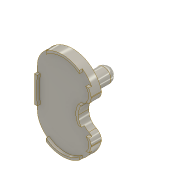
# Autodesk Inventor part: 1
Saved by Autodesk Inventor 2017 (Build 210142000, 142)
## iProperties
Created: 2020-04-05
Part Number: 1
Material: Tytan 6Al-4V
Document SubType Name: Modeling
Designer: Kinga Nowak
Density: 4.43 g/cm^3
Appearance: Tytan — polerowany
Authority: dr Marta Kiel-Jamrozik
Checked By: dr Marta Kiel-Jamrozik
Mfg Approved By: dr Marta Kiel-Jarmozik
Description: Endoproteza stawu kolanowego
Project: część piszczelowa
Author: Kinga Nowak
Autodesk Inventor part; units mm, degrees
ref_plane "YZ Plane" through (0, 0, 0) normal (1, 0, 0) x (0, 1, 0)
ref_plane "XZ Plane" through (0, 0, 0) normal (0, 1, 0) x (-1, 0, 0)
sketch "Szkic1" plane through (0, 0, 0) normal (0, 1, 0) x (-1, 0, 0)
  line L0 (-4, -50.1202) -> (-4, -37.2024)
  line L1 (-42.5, -51.8732) -> (-42.5, -51.3513)
  line L2 (-4, -38) -> (-4, -50.1202)
  arc A0 (-38.9822, -45.8888) -> (-34, -38.0004) centre (-42.4987, -38.1503) ccw
  line L3 (-42.5, -51.3513) -> (-42.5, -51.8732)
  arc A1 (-34, -38.0004) -> (-34.0517, -37.2023) centre (-42.4987, -38.1503) ccw
  arc A2 (-38.9822, -45.8888) -> (-42.5, -51.3513) centre (-36.5, -51.3513) ccw
  arc A3 (-42.5, -51.8732) -> (-6.8354, -58.8964) centre (-23.0549, -47.1948) ccw
  arc A4 (-6.8354, -58.8964) -> (-4, -50.1202) centre (-19, -50.1202) ccw
  line L4 (-42.5, -51.3513) -> (-42.5, -51.8732)
  line L5 (-4, -24.2847) -> (-4, -37.2024)
  line L6 (-42.5, -22.5011) -> (-42.5, -23.0533)
  line L7 (-4, -36.4049) -> (-4, -24.2847)
  arc A5 (-34, -36.4047) -> (-38.9822, -28.5157) centre (-42.4987, -36.2542) ccw
  line L8 (-42.5, -23.0533) -> (-42.5, -22.5011)
  arc A6 (-34.0517, -37.2023) -> (-34, -36.4047) centre (-42.4987, -36.2542) ccw
  arc A7 (-42.5, -23.0533) -> (-38.9822, -28.5157) centre (-36.5, -23.0533) ccw
  arc A8 (-6.8187, -15.5316) -> (-42.5, -22.5011) centre (-23.0604, -27.2024) ccw
  arc A9 (-4, -24.2847) -> (-6.8187, -15.5316) centre (-19, -24.2847) ccw
  line L9 (-42.5, -23.0533) -> (-42.5, -22.5011)
  line L10 (-12, -10.5391) -> (-12, -12.5391)
  line L11 (-34.5, -10.7971) -> (-34.5, -12.7971)
  arc A10 (-12, -12.5391) -> (-34.5, -12.7971) centre (-23.0889, -26.7178) ccw
  line L12 (-11.9997, -63.8616) -> (-11.9997, -61.8657)
  line L13 (-34.5004, -63.596) -> (-34.5004, -61.6077)
  arc A11 (-34.5004, -61.6077) -> (-11.9997, -61.8657) centre (-23.0889, -47.6872) ccw
  line L14 (-35.8952, -43.5023) -> (-33.8952, -43.5023)
  line L15 (-35.8952, -30.9023) -> (-33.8952, -30.9023)
  arc A12 (-33.8952, -43.5023) -> (-33.8952, -30.9023) centre (-44.1084, -37.2023) ccw
  line L16 (-4, -28) -> (-6, -28)
  line L17 (-6, -46) -> (-4, -46)
  arc A13 (-6, -46) -> (-6, -28) centre (-89.405, -37) ccw
  line L18 (-40.8175, -18) -> (-38.8175, -18)
  line L19 (-40.8176, -27.2196) -> (-38.8176, -27.2198)
  arc A14 (-38.8175, -18) -> (-38.9822, -27.2198) centre (-34.316, -22.6918) ccw
  line L20 (-41.0122, -56.0002) -> (-39.0216, -56.0002)
  line L21 (-39.0216, -56.0002) -> (-41.0122, -56.0002)
  line L22 (-41.0216, -47.4073) -> (-39.0216, -47.4076)
  arc A15 (-39.0216, -47.4076) -> (-39.0216, -56.0002) centre (-35.5308, -51.7039) ccw
  line L23 (-19, -7.6189) -> (11, -7.6189) construction
  point P0 (0, 0)
  point P1 (-42.5001, -29.6503)
  point P2 (-4, -22.2491)
  point P3 (-23.0549, -67.1948)
  point P4 (-23.0549, -67.1948)
  point P5 (-42.5, -44.7542)
  point P6 (-23.0604, -7.2024)
  point P7 (-23.0604, -7.2024)
  dimension "d12" = 15
  dimension "d13" = 30
  dimension "d14" = 6
  dimension "d15" = 20
  dimension "d21" = 38.5
  dimension "d53" = 2
  constraints: 49 point on circle, 48 end point, 16 centre point, 4 horizontal, 4 point on line, 4 tangent, 4 vertical, 2 coincident, 2 parallel, 1 collinear, 1 perpendicular, 5 other
  measures "d12" radius of A4
  measures "d13" distance from line of L0 A0.end
  measures "d14" radius of A2
  measures "d15" radius of A3
  measures "d21" distance from line of L1.end L2
  measures "d53" distance of L18.start L18.end
extrude "Wyciągnięcie proste1" add sketch "Szkic1" along normal blind 5
extrude "Wyciągnięcie proste2" add sketch "Szkic1" against normal blind 2 contours L17 A13 L16 L5 L0 | A3 L13 A11 L12 | A3 L1 A2 L22 A15 L20 | L10 A10 L11 A8 | L18 A14 L19 A7 L6 A8 | A0 A1 A6 A5 L15 A12 L14
sketch "Szkic5" plane through (0, 5, 0) normal (0, 1, 0) x (1, 0, 0)
  line L0 (4, 28) -> (6, 28) projected
  arc A0 (6, 46) -> (6, 28) centre (89.405, 37) ccw projected
  line L1 (6, 46) -> (4, 46) projected
  line L2 (4, 50.1202) -> (4, 46) projected
  arc A1 (6.8354, 58.8964) -> (4, 50.1202) centre (19, 50.1202) ccw projected
  arc A2 (11.9997, 63.8616) -> (6.8354, 58.8964) centre (23.0549, 47.1948) ccw projected
  line L3 (11.9997, 63.8616) -> (11.9997, 61.8657) projected
  arc A3 (34.5004, 61.6077) -> (11.9997, 61.8657) centre (23.0889, 47.6872) ccw projected
  line L4 (34.5004, 61.6077) -> (34.5004, 63.596) projected
  arc A4 (41.0122, 56.0002) -> (34.5004, 63.596) centre (23.0549, 47.1948) ccw projected
  line L5 (41.0122, 56.0002) -> (39.0216, 56.0002) projected
  arc A5 (39.0216, 47.4076) -> (39.0216, 56.0002) centre (35.5308, 51.7039) ccw projected
  line L6 (39.0216, 47.4076) -> (41.0216, 47.4073) projected
  arc A6 (38.9822, 45.8888) -> (41.0216, 47.4073) centre (36.5, 51.3513) ccw projected
  arc A7 (38.9822, 45.8888) -> (35.8952, 43.5023) centre (42.4987, 38.1503) ccw projected
  line L7 (35.8952, 43.5023) -> (33.8952, 43.5023) projected
  arc A8 (33.8952, 43.5023) -> (33.8952, 30.9023) centre (44.1084, 37.2023) ccw projected
  line L8 (33.8952, 30.9023) -> (35.8952, 30.9023) projected
  arc A9 (35.8952, 30.9023) -> (38.9822, 28.5157) centre (42.4987, 36.2542) ccw projected
  arc A10 (40.8176, 27.2196) -> (38.9822, 28.5157) centre (36.5, 23.0533) ccw projected
  line L9 (40.8176, 27.2196) -> (38.9822, 27.2198) projected
  arc A11 (38.8175, 18) -> (38.9822, 27.2198) centre (34.316, 22.6918) ccw projected
  line L10 (38.8175, 18) -> (40.8175, 18) projected
  arc A12 (34.5, 10.7971) -> (40.8175, 18) centre (23.0604, 27.2024) ccw projected
  line L11 (34.5, 10.7971) -> (34.5, 12.7971) projected
  arc A13 (12, 12.5391) -> (34.5, 12.7971) centre (23.0889, 26.7178) ccw projected
  line L12 (12, 12.5391) -> (12, 10.5391) projected
  arc A14 (6.8187, 15.5316) -> (12, 10.5391) centre (23.0604, 27.2024) ccw projected
  arc A15 (4, 24.2847) -> (6.8187, 15.5316) centre (19, 24.2847) ccw projected
  line L13 (4, 28) -> (4, 24.2847) projected
  arc A16 (12, 10.5391) -> (34.5, 10.7971) centre (23.0604, 27.2024) ccw projected
  arc A17 (34.5004, 63.596) -> (11.9997, 63.8616) centre (23.0549, 47.1948) ccw projected
  line L14 (4, 28) -> (4, 46) projected
  arc A18 (40.8175, 18) -> (42.5, 22.5011) centre (23.0604, 27.2024) ccw projected
  arc A19 (42.5, 23.0533) -> (40.8176, 27.2196) centre (36.5, 23.0533) ccw projected
  line L15 (42.5, 23.0533) -> (42.5, 22.5011) projected
  arc A20 (34.0517, 37.2023) -> (35.8952, 30.9023) centre (42.4987, 36.2542) ccw projected
  arc A21 (35.8952, 43.5023) -> (34.0517, 37.2023) centre (42.4987, 38.1503) ccw projected
  arc A22 (42.5, 51.8732) -> (41.0122, 56.0002) centre (23.0549, 47.1948) ccw projected
  line L16 (42.5, 51.8732) -> (42.5, 51.3513) projected
  arc A23 (41.0216, 47.4073) -> (42.5, 51.3513) centre (36.5, 51.3513) ccw projected
  arc A24 (6.8187, 15.5316) -> (42.5, 22.5011) centre (23.0604, 27.2024) ccw projected
  line L17 (20.4612, 7.372) -> (50.4612, 7.372) construction
  line L18 (4, 50.1202) -> (4, 24.2847) projected
  circle A25 centre (19, 37.372) radius 10
  dimension "d74" = 20
  constraints: 2 end point, 2 point on circle, 1 centre point, 1 horizontal
  measures "d74" diameter of A25
ref_plane "Płaszczyzna konstrukcyjna1" through (0, 20, 0) normal (0, 1, 0) x (1, 0, 0)
sketch "Szkic6" plane through (0, 20, 0) normal (0, 1, 0) x (1, 0, 0)
  circle A0 centre (19, 37.372) radius 5
  point P0 (0, 0)
  dimension "d76" = 10
  constraints: 1 centre point, 1 coincident
  measures "d76" diameter of A0
loft "Wyciągnięcie złożone1" add profiles "Szkic6", "Szkic5" contours all / A25
sketch "Szkic7" plane through (19, 20, -37.372) normal (0, 1, 0) x (1, 0, 0)
  circle A0 centre (0, 0) radius 5
  point P0 (-19, -37.372)
  dimension "d85" = 10
  constraints: 1 centre point
  measures "d85" diameter of A0
extrude "Wyciągnięcie proste3" add sketch "Szkic7" along normal blind 15
fillet "Zaokrąglenie1" radius 5 1 edges at (14, 35, -37.372)
